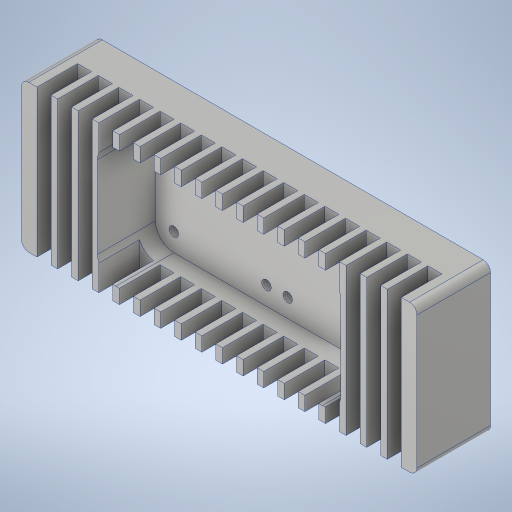
# Autodesk Inventor part: Heat sink
Saved by Autodesk Inventor 2023.4 (Build 274418000, 418)
## iProperties
Created: 2025-01-05
Part Number: Heat sink
Material: Aluminum 6061
Document SubType Name: Modeling
Designer: jmcintyr
Density: 2.7 g/cm^3
Appearance: Aluminum - Flat
Author: jmcintyr
Autodesk Inventor part; units mm, degrees
ref_plane "YZ Plane" through (0, 0, 0) normal (1, 0, 0) x (0, 1, 0)
ref_plane "XZ Plane" through (0, 0, 0) normal (0, 1, 0) x (-1, 0, 0)
ref_plane "XY Plane" through (0, 0, 0) normal (0, 0, 1) x (1, 0, 0)
sketch "Sketch1" plane through (0, 0, 0) normal (0, 0, 1) x (1, 0, 0)
  line L0 (0, 0) -> (136.525, 0)
  line L1 (136.525, 0) -> (136.525, 50.8)
  line L2 (136.525, 50.8) -> (0, 50.8)
  line L3 (0, 50.8) -> (0, 0)
  dimension "d0" = 136.525
  dimension "d1" = 50.8
  constraints: 8 end point, 2 parallel, 1 horizontal, 1 perpendicular
  measures "d0" distance of L2.end L1.end
  measures "d1" distance of L1.end L0.end
extrude "Extrusion1" add sketch "Sketch1" against normal blind 25.4
sketch "Sketch2" plane through (0, 0, 0) normal (0, 0, 1) x (1, 0, 0)
  line L0 (26.2625, 45.9) -> (110.2625, 45.9)
  line L1 (110.2625, 45.9) -> (110.2625, 4.9)
  line L2 (110.2625, 4.9) -> (26.2625, 4.9)
  line L3 (26.2625, 4.9) -> (26.2625, 45.9)
  line L4 (26.2625, 45.9) -> (110.2625, 4.9) construction
  line L5 (110.2625, 45.9) -> (26.2625, 4.9) construction
  line L6 (136.525, 50.8) -> (0, 50.8) projected
  line L7 (136.525, 0) -> (136.525, 50.8) projected
  point P0 (0, 0)
  point P1 (68.2625, 25.4)
  point P2 (68.2625, 50.8)
  point P3 (136.525, 25.4)
  dimension "d4" = 84
  dimension "d5" = 41
  constraints: 12 end point, 4 midpoint, 2 parallel, 1 horizontal, 1 horizontal alignment, 1 perpendicular, 1 vertical alignment
  measures "d4" distance of L1.end L2.end
  measures "d5" distance of L0.end L1.end
extrude "Extrusion2" cut sketch "Sketch2" against normal blind 20
fillet "Fillet1" radius 6.35 4 edges at (26.2625, 4.9, -10) (26.2625, 45.9, -10) (110.2625, 45.9, -10) (110.2625, 4.9, -10)
sketch "Sketch4" plane through (0, 0, -20) normal (0, 0, 1) x (1, 0, 0)
  arc A0 (103.9125, 4.9) -> (110.2625, 11.25) centre (103.9125, 11.25) ccw projected
  line L0 (110.2625, 39.55) -> (110.2625, 11.25) projected
  arc A1 (110.2625, 39.55) -> (103.9125, 45.9) centre (103.9125, 39.55) ccw projected
  line L1 (32.6125, 45.9) -> (103.9125, 45.9) projected
  arc A2 (32.6125, 45.9) -> (26.2625, 39.55) centre (32.6125, 39.55) ccw projected
  line L2 (26.2625, 11.25) -> (26.2625, 39.55) projected
  arc A3 (26.2625, 11.25) -> (32.6125, 4.9) centre (32.6125, 11.25) ccw projected
  line L3 (103.9125, 4.9) -> (32.6125, 4.9) projected
  point P0 (0, 0)
  point P1 (64.6125, 39.55)
  point P2 (64.6125, 11.25)
  point P3 (71.9125, 11.25)
  point P4 (71.9125, 39.55)
  dimension "d9" = 32
  dimension "d10" = 32
  dimension "d11" = 32
  dimension "d12" = 32
  constraints: 4 horizontal alignment
  measures "d9" distance of point (64.612, 39.55) A2.centre
  measures "d10" distance of point (71.912, 39.55) A1.centre
  measures "d11" distance of A0.centre point (71.912, 11.25)
  measures "d12" distance of A3.centre point (64.612, 11.25)
hole "Hole1" at (64.6125, 39.55, -20) at (64.6125, 11.25, -20) at (71.9125, 11.25, -20) at (71.9125, 39.55, -20) at (32.6125, 39.55, -20) at (32.6125, 11.25, -20) at (103.9125, 11.25, -20) at (103.9125, 39.55, -20) direction (0, 0, -1) diameter 3.302 end through all thread size "8-32 UNC" class "2B" standard "ANSI Unified Screw Threads"
sketch "Sketch5" plane through (0, 0, 0) normal (0, 0, 1) x (1, 0, 0)
  line L0 (0, 50.8) -> (0, 0) projected
  line L1 (5.3848, 50.8) -> (5.3848, 0)
  line L2 (10.2108, 50.8) -> (10.2108, 0)
  line L3 (5.3848, 50.8) -> (10.2108, 50.8)
  line L4 (136.525, 50.8) -> (0, 50.8) projected
  line L5 (10.2108, 0) -> (5.3848, 0)
  line L6 (0, 0) -> (136.525, 0) projected
  dimension "d20" = 5.3848
  dimension "d21" = 4.826
  constraints: 8 end point, 2 collinear, 2 parallel
  measures "d20" distance between parallel lines of L0 L1
  measures "d21" distance between parallel lines of L1 L2
extrude "Extrusion3" cut sketch "Sketch5" against normal blind 14 contours L3 L2 L5 L1
pattern_linear "Rectangular Pattern1" count 18 spacing 7.112 along (1, 0, 0) of "Extrusion3"
fillet "Fillet2" radius 2.54 4 edges at (0, 0, -12.7) (136.525, 0, -12.7) (136.525, 50.8, -12.7) (0, 50.8, -12.7)
body "Solid1"
